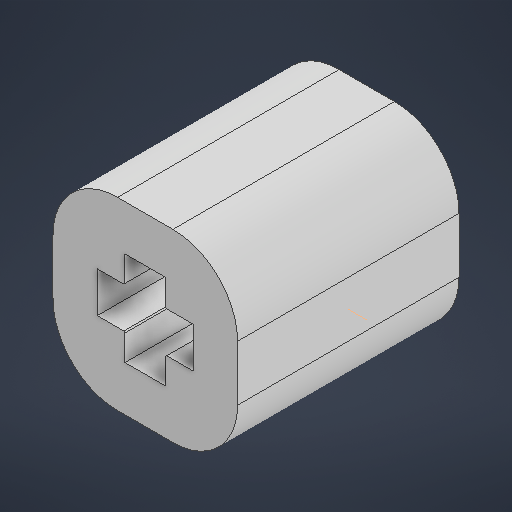
# Autodesk Inventor part: Acoplador
Saved by Autodesk Inventor 2026.2 (Build 302298010, 298A)
## iProperties
Created: 2026-04-17
Part Number: Acoplador
Material: Genérico
Document SubType Name: Modeling
Designer: Jose Carlos
Density: 1 g/cm^3
Appearance: Valor por defecto
Author: Jose Carlos
Autodesk Inventor part; units mm, degrees
ref_plane "YZ Plane" through (0, 0, 0) normal (1, 0, 0) x (0, 1, 0)
ref_plane "XZ Plane" through (0, 0, 0) normal (0, 1, 0) x (-1, 0, 0)
ref_plane "XY Plane" through (0, 0, 0) normal (0, 0, 1) x (1, 0, 0)
sketch "Boceto2" plane through (0, 0, 0) normal (0, 0, 1) x (1, 0, 0)
  circle A0 centre (0, 0) radius 1.6
  line L0 (1.1, -2.55) -> (-1.1, -2.55)
  line L1 (-1.1, -2.55) -> (-1.1, 2.55)
  line L2 (-1.1, 2.55) -> (1.1, 2.55)
  line L3 (1.1, 2.55) -> (1.1, -2.55)
  line L4 (1.1, -2.55) -> (-1.1, 2.55) construction
  line L5 (-1.1, -2.55) -> (1.1, 2.55) construction
  line L6 (-2.6, -1.1) -> (2.6, -1.1)
  line L7 (2.6, -1.1) -> (2.6, 1.1)
  line L8 (2.6, 1.1) -> (-2.6, 1.1)
  line L9 (-2.6, 1.1) -> (-2.6, -1.1)
  line L10 (-2.6, -1.1) -> (2.6, 1.1) construction
  line L11 (2.6, -1.1) -> (-2.6, 1.1) construction
  line L12 (5, -5) -> (-5, -5)
  line L13 (-5, -5) -> (-5, 5)
  line L14 (-5, 5) -> (5, 5)
  line L15 (5, 5) -> (5, -5)
  line L16 (5, -5) -> (-5, 5) construction
  line L17 (-5, -5) -> (5, 5) construction
  point P0 (-1.1, -1.1619)
  point P1 (-1.1619, -1.1)
  point P2 (-1.1619, 1.1)
  point P3 (-1.1, 1.1619)
  point P4 (1.1, 1.1619)
  point P5 (1.1619, 1.1)
  point P6 (1.1619, -1.1)
  point P7 (1.1, -1.1619)
  dimension "d0" = 3.2
  dimension "d1" = 2.2
  dimension "d2" = 5.1
  dimension "d3" = 2.2
  dimension "d4" = 5.2
  dimension "d5" = 10
  dimension "d6" = 10
  constraints: 36 end point, 6 midpoint, 6 parallel, 3 horizontal, 3 perpendicular, 1 centre point, 1 coincident
  measures "d0" diameter of A0
  measures "d1" distance of L1.end L2.end
  measures "d2" distance of L0.end L1.end
  measures "d3" distance of L6.end L7.end
  measures "d4" distance of L7.end L8.end
  measures "d5" distance of L12.end L13.end
  measures "d6" distance of L13.end L14.end
extrude "Extrusión1" add sketch "Boceto2" along normal mid plane 12
fillet "Empalme1" radius 3.5 4 edges at (5, 5, 0) (-5, 5, 0) (5, -5, 0) (-5, -5, 0)
